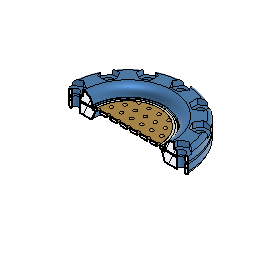
Microphone Capsule (Autodesk Fusion 360 design; units mm, degrees)
Autodesk Fusion 360 part; units mm, degrees
note: some values were not read from the file. Chosen so that the rebuilt part matches the saved one: which face or edge a step refers to. Set by a fixed rule: which sketch regions a step uses.
ref_plane "WorkPlane1" through (0, 0, -5) normal (0, 0, 1) x (1, 0, 0)
sketch "Top" plane through (0, 0, -5) normal (0, 0, 1) x (1, 0, 0)
  circle A0 centre (0, 0) radius 10.5
  circle A1 centre (0, 15.5) radius 1.175
  line L0 (0, 0) -> (0, 15.5) construction
  circle A2 centre (0, 0) radius 17.475
  circle A3 centre (0, 15.5) radius 1.975 construction
  circle A4 centre (-7.75, 13.4234) radius 1.175
  circle A5 centre (-13.4234, 7.75) radius 1.175
  circle A6 centre (-15.5, 0) radius 1.175
  circle A7 centre (-13.4234, -7.75) radius 1.175
  circle A8 centre (-7.75, -13.4234) radius 1.175
  circle A9 centre (0, -15.5) radius 1.175
  circle A10 centre (7.75, -13.4234) radius 1.175
  circle A11 centre (13.4234, -7.75) radius 1.175
  circle A12 centre (15.5, 0) radius 1.175
  circle A13 centre (13.4234, 7.75) radius 1.175
  circle A14 centre (7.75, 13.4234) radius 1.175
  circle A15 centre (0, 0) radius 11.4
  circle A16 centre (0, 0) radius 9.7
  line L1 (-1.1836, 13.45) -> (-2.3671, 15.5)
  line L2 (-2.3671, 15.5) -> (-1.1836, 17.55)
  line L3 (-1.1836, 17.55) -> (1.1836, 17.55)
  line L4 (1.1836, 17.55) -> (2.3671, 15.5)
  line L5 (2.3671, 15.5) -> (1.1836, 13.45)
  line L6 (-1.1836, 13.45) -> (1.1836, 13.45)
  circle A17 centre (0, 15.5) radius 2.05 construction
  line L7 (-7.75, 15.7905) -> (-5.7, 14.607)
  line L8 (-9.8, 14.607) -> (-7.75, 15.7905)
  line L9 (-9.8, 12.2398) -> (-9.8, 14.607)
  line L10 (-7.75, 11.0563) -> (-9.8, 12.2398)
  line L11 (-7.75, 11.0563) -> (-5.7, 12.2398)
  line L12 (-5.7, 14.607) -> (-5.7, 12.2398)
  line L13 (-14.607, 9.8) -> (-12.2398, 9.8)
  line L14 (-15.7905, 7.75) -> (-14.607, 9.8)
  line L15 (-14.607, 5.7) -> (-15.7905, 7.75)
  line L16 (-12.2398, 5.7) -> (-14.607, 5.7)
  line L17 (-12.2398, 5.7) -> (-11.0563, 7.75)
  line L18 (-12.2398, 9.8) -> (-11.0563, 7.75)
  line L19 (-17.55, 1.1836) -> (-15.5, 2.3671)
  line L20 (-17.55, -1.1836) -> (-17.55, 1.1836)
  line L21 (-15.5, -2.3671) -> (-17.55, -1.1836)
  line L22 (-13.45, -1.1836) -> (-15.5, -2.3671)
  line L23 (-13.45, -1.1836) -> (-13.45, 1.1836)
  line L24 (-15.5, 2.3671) -> (-13.45, 1.1836)
  line L25 (-15.7905, -7.75) -> (-14.607, -5.7)
  line L26 (-14.607, -9.8) -> (-15.7905, -7.75)
  line L27 (-12.2398, -9.8) -> (-14.607, -9.8)
  line L28 (-11.0563, -7.75) -> (-12.2398, -9.8)
  line L29 (-11.0563, -7.75) -> (-12.2398, -5.7)
  line L30 (-14.607, -5.7) -> (-12.2398, -5.7)
  line L31 (-9.8, -14.607) -> (-9.8, -12.2398)
  line L32 (-7.75, -15.7905) -> (-9.8, -14.607)
  line L33 (-5.7, -14.607) -> (-7.75, -15.7905)
  line L34 (-5.7, -12.2398) -> (-5.7, -14.607)
  line L35 (-5.7, -12.2398) -> (-7.75, -11.0563)
  line L36 (-9.8, -12.2398) -> (-7.75, -11.0563)
  line L37 (-1.1836, -17.55) -> (-2.3671, -15.5)
  line L38 (1.1836, -17.55) -> (-1.1836, -17.55)
  line L39 (2.3671, -15.5) -> (1.1836, -17.55)
  line L40 (1.1836, -13.45) -> (2.3671, -15.5)
  line L41 (1.1836, -13.45) -> (-1.1836, -13.45)
  line L42 (-2.3671, -15.5) -> (-1.1836, -13.45)
  line L43 (7.75, -15.7905) -> (5.7, -14.607)
  line L44 (9.8, -14.607) -> (7.75, -15.7905)
  line L45 (9.8, -12.2398) -> (9.8, -14.607)
  line L46 (7.75, -11.0563) -> (9.8, -12.2398)
  line L47 (7.75, -11.0563) -> (5.7, -12.2398)
  line L48 (5.7, -14.607) -> (5.7, -12.2398)
  line L49 (14.607, -9.8) -> (12.2398, -9.8)
  line L50 (15.7905, -7.75) -> (14.607, -9.8)
  line L51 (14.607, -5.7) -> (15.7905, -7.75)
  line L52 (12.2398, -5.7) -> (14.607, -5.7)
  line L53 (12.2398, -5.7) -> (11.0563, -7.75)
  line L54 (12.2398, -9.8) -> (11.0563, -7.75)
  line L55 (17.55, -1.1836) -> (15.5, -2.3671)
  line L56 (17.55, 1.1836) -> (17.55, -1.1836)
  line L57 (15.5, 2.3671) -> (17.55, 1.1836)
  line L58 (13.45, 1.1836) -> (15.5, 2.3671)
  line L59 (13.45, 1.1836) -> (13.45, -1.1836)
  line L60 (15.5, -2.3671) -> (13.45, -1.1836)
  line L61 (15.7905, 7.75) -> (14.607, 5.7)
  line L62 (14.607, 9.8) -> (15.7905, 7.75)
  line L63 (12.2398, 9.8) -> (14.607, 9.8)
  line L64 (11.0563, 7.75) -> (12.2398, 9.8)
  line L65 (11.0563, 7.75) -> (12.2398, 5.7)
  line L66 (14.607, 5.7) -> (12.2398, 5.7)
  line L67 (9.8, 14.607) -> (9.8, 12.2398)
  line L68 (7.75, 15.7905) -> (9.8, 14.607)
  line L69 (5.7, 14.607) -> (7.75, 15.7905)
  line L70 (5.7, 12.2398) -> (5.7, 14.607)
  line L71 (5.7, 12.2398) -> (7.75, 11.0563)
  line L72 (9.8, 12.2398) -> (7.75, 11.0563)
  circle A18 centre (0, 0) radius 10.6
  point P0 (0, 10.5)
  dimension "d2" = 21
  dimension "d3" = 2.35
  dimension "d7" = 0.8
  dimension "d9" = 360
  dimension "d35" = 4.1
  dimension "d62" = 0.8
  dimension "d63" = 0.1
  dimension "d82" = 5
  dimension "d83" = 0.8
  constraint coincident A0.centre L0.start
  constraint vertical L0
  constraint coincident A1.centre L0.end
  constraint concentric A0 A2
  constraint concentric A1 A3
  constraint tangent A2 A3
  constraint concentric A0 A15
  constraint perpendicular L0 L6
  constraint equal L5 L6
  constraint equal L4 L5
  constraint equal L3 L4
  constraint equal L2 L3
  constraint equal L1 L2
  constraint concentric A1 A17
  constraint tangent L5 A17
  constraint tangent L4 A17
  constraint tangent L3 A17
  constraint tangent L2 A17
  constraint tangent L1 A17
  constraint parallel L2 L5
  constraint concentric A16 A18
  constraint coincident A0 P0
  constraint coincident L0 P0
  measures "d2" diameter of A0
  measures "d3" diameter of A1
  measures "d7" distance of A1 A3
  measures "d35" distance of L2.end L6
  measures "d62" distance of A0 A16
  measures "d63" distance of A0 A18
  measures "d82" distance of A1.centre P0
  measures "d83" distance of A15 A18
ref_plane "WorkPlane2" through (0, -41, 0) normal (0, 1, 0) x (0, 0, 1)
sketch "Side" plane through (0, -41, 0) normal (0, 1, 0) x (1, 0, 0)
  line L0 (-17.475, 5) -> (17.475, 5)
  line L1 (-10.5, 5) -> (10.5, 5)
  line L2 (-11.4, 5) -> (11.4, 5)
  line L3 (17.475, -2.6) -> (17.475, -0.766)
  line L4 (17.475, -3.2) -> (10.75, -3.2)
  line L5 (12.95, -6.2) -> (16.475, -6.2)
  line L6 (17.475, -5.2) -> (17.475, -3.2)
  line L7 (17.475, 5) -> (17.475, 0) construction
  line L8 (10.5, 5) -> (10.5, -2.7) construction
  line L9 (17.1178, 0) -> (10.6827, 0)
  line L10 (10.6827, 0) -> (9.7, -2.7)
  line L11 (10.5, -3) -> (11.4, -3)
  line L12 (0, 0) -> (10.6827, 0) construction
  line L13 (0, 0) -> (0, 5) construction
  line L14 (-9.7, 5) -> (9.7, 5)
  line L15 (9.7, 5) -> (9.7, -2.7) construction
  line L16 (11.4, 5) -> (11.4, -3) construction
  line L17 (10.5, -3) -> (10.5, -2.7)
  line L18 (10.5, -2.7) -> (9.7, -2.7)
  line L19 (11.4, -3) -> (17.475, -3) construction
  line L20 (-10.6, 5) -> (10.6, 5)
  line L21 (10.6, 5) -> (10.6, -3.4598) construction
  line L22 (11.4, -3) -> (17.475, -2.6)
  arc A0 (16.475, -6.2) -> (17.475, -5.2) centre (16.475, -5.2) ccw
  arc A1 (17.475, -0.766) -> (17.1178, 0) centre (16.475, -0.766) ccw
  line L23 (17.1178, 0) -> (17.475, -0.2997) construction
  line L24 (17.475, -0.2997) -> (17.475, -0.766) construction
  line L25 (13.45, 5) -> (13.45, -6.2) construction
  arc A2 (10.75, -3.2) -> (10.6, -3.4598) centre (10.9, -3.4598) ccw
  arc A3 (10.6, -3.4598) -> (12.95, -6.2) centre (13.3726, -3.4598) ccw
  line L26 (10.75, -3.2) -> (10.6, -3.2866) construction
  point P0 (17.475, -6.2)
  point P1 (17.475, -2.6)
  point P2 (17.475, -4.6)
  point P3 (13.45, 5)
  point P4 (17.55, 5)
  dimension "d13" = 3
  dimension "d16" = 3
  dimension "d31" = 0.3
  dimension "d37" = 1.6
  dimension "d85" = 0.4
  dimension "d91" = 70
  dimension "d92" = 1
  dimension "d93" = 40
  dimension "d95" = 1
  dimension "d96" = 0.5
  dimension "d97" = 0.3
  dimension "d98" = 30
  dimension "d99" = 0.2
  constraint coincident L0.end L7.start
  constraint coincident L1.end L8.start
  constraint perpendicular L0 L8
  constraint perpendicular L0 L7
  constraint collinear L3 L6
  constraint collinear L3 L7
  constraint parallel L0 L9
  constraint parallel L9 L11
  constraint parallel L4 L11
  constraint coincident L12.start L13.start
  constraint collinear L9 L12
  constraint parallel L4 L5
  constraint midpoint L1 L13.end
  constraint coincident L14.end L15.start
  constraint perpendicular L0 L15
  constraint coincident L2.end L16.start
  constraint perpendicular L0 L16
  constraint perpendicular L11 L17
  constraint collinear L8 L17
  constraint coincident L6 P2
  constraint coincident L3 L19.end
  constraint perpendicular L3 L19
  constraint coincident L20.end L21.start
  constraint perpendicular L0 L21
  constraint coincident L8.end L17.end
  constraint coincident L7.end L9
  constraint coincident L7.end L3
  constraint coincident L3 P1
  constraint coincident P1 L22
  constraint coincident P0 L6
  constraint coincident P0 L5
  constraint tangent L6 A0
  constraint tangent L5 A0
  constraint coincident L9.end L10
  constraint coincident L10.start L9
  constraint coincident L10.end L15.end
  constraint parallel L9 L18
  constraint coincident L9.end L10.start
  constraint tangent L3 A1
  constraint coincident L9.start A1.end
  constraint tangent A1 L23
  constraint collinear L3 L24
  constraint coincident P3 L25.start
  constraint perpendicular L0 L25
  constraint coincident P1 L3.start
  constraint coincident L5 L25.end
  constraint tangent A2 A3
  constraint coincident L21.end A2.end
  constraint tangent L21 A3
  constraint coincident L4.end A2.start
  constraint tangent A2 L26
  constraint coincident L21 L26.end
  measures "d13" distance of L11.end L9
  measures "d16" distance of L4 P0
  measures "d31" distance of L11.start L8.end
  measures "d37" distance of L5 P2
  measures "d85" distance of L11 P1
  measures "d91" angle of L9 L10
  measures "d92" radius of A1
  measures "d93" angle of L9 L23
  measures "d95" radius of A0
  measures "d96" distance of L5.start L25
  measures "d97" radius of A2
  measures "d98" angle of L4 L26
  measures "d99" distance of L11 L4.end
ref_plane "WorkPlane3" through (0, 0, 0) normal (0, 1, 0) x (0, 0, 1)
sketch "Sketch3" plane through (0, 0, 0) normal (0, 1, 0) x (1, 0, 0)
  arc A0 (16.475, -6.2) -> (17.475, -5.2) centre (16.475, -5.2) ccw
  line L0 (12.95, -6.2) -> (16.475, -6.2)
  line L1 (17.475, -3.2) -> (10.75, -3.2)
  line L2 (17.475, -5.2) -> (17.475, -3.2)
  line L3 (17.475, -2.6) -> (17.475, -0.766)
  line L4 (11.4, -3) -> (17.475, -2.6)
  line L5 (10.5, -3) -> (11.4, -3)
  line L6 (10.5, -3) -> (10.5, -2.7)
  line L7 (10.5, -2.7) -> (9.7, -2.7)
  line L8 (10.6827, 0) -> (9.7, -2.7)
  line L9 (17.1178, 0) -> (10.6827, 0)
  arc A1 (17.475, -0.766) -> (17.1178, 0) centre (16.475, -0.766) ccw
  arc A2 (10.75, -3.2) -> (10.6, -3.4598) centre (10.9, -3.4598) ccw
  arc A3 (10.6, -3.4598) -> (12.95, -6.2) centre (13.3726, -3.4598) ccw
revolve "Revolve1" add sketch "Sketch3" angle 360 about axis through (0, 0, -4.7808) along (0, 0, 1) makes body 1 at (14.8693, -1.3812, 0) makes body 2 at (15.1283, -1.4022, 3.2)
extrude "Extrude3" cut sketch "Top" against normal up to surface (6.2 mm away) from surface at 11.2 contours A1 | A4 | A5 | A6 | A7 | A8 | A9 | A10 | A11 | A12 | A13 | A14 bodies 1 2
extrude "Extrude5" cut sketch "Top" against normal up to surface (1.6 mm away) from surface at 11.2 contours A2 L55 L57 L58 L59 L60 | A2 L55 L56 L57 | A2 L61 L63 L64 L65 L66 | A2 L61 L62 L63 | A2 L49 L50 L51 | A2 L49 L51 L52 L53 L54 | A2 L67 L69 L70 L71 L72 | A2 L67 L68 L69 | A2 L43 L44 L45 | A2 L43 L45 L46 L47 L48 | A2 L1 L2 L4 L5 L6 | A2 L2 L3 L4 | A2 L37 L38 L39 | A2 L37 L39 L40 L41 L42 | A2 L7 L9 L10 L11 L12 | A2 L7 L8 L9 | A2 L31 L32 L33 | A2 L31 L33 L34 L35 L36 | A2 L13 L15 L16 L17 L18 | A2 L13 L14 L15 | A2 L25 L26 L27 | A2 L25 L27 L28 L29 L30 | A2 L19 L21 L22 L23 L24 | A2 L19 L20 L21 bodies 2
ref_plane "WorkPlane1" through (0, 0, -10) normal (0, 0, 1) x (1, 0, 0) in component "Brass Base Plate"
sketch "Sketch1" plane through (0, 0, -10) normal (0, 0, 1) x (1, 0, 0) in component "Brass Base Plate"
  circle A0 centre (0, 0) radius 17.475 construction
  circle A1 centre (0, 0) radius 10.2
  line L0 (0, 10.2) -> (0, -10.2) construction
  arc A2 (-8.8335, 5.1) -> (8.8335, 5.1) centre (0, 10.2) ccw construction
  line L1 (8.8335, 5.1) -> (-8.8335, -5.1) construction
  line L2 (-8.8335, 5.1) -> (8.8335, -5.1) construction
  line L3 (0, 10.2) -> (8.8335, -5.1) construction
  line L4 (0, 10.2) -> (-8.8335, -5.1) construction
  line L5 (-9.8761, 2.55) -> (9.8761, 2.55) construction
  line L6 (8.8335, -5.1) -> (-8.8335, -5.1) construction
  line L7 (8.8335, 5.1) -> (0, -10.2) construction
  line L8 (9.9984, -2.0178) -> (3.2518, 9.6678) construction
  line L9 (-2.7297, 9.828) -> (7.1464, -7.278) construction
  circle A3 centre (4.4167, 2.55) radius 0.5
  circle A4 centre (5.889, 0) radius 0.5
  circle A5 centre (1.4722, 2.55) radius 0.5
  line L10 (9.9984, 2.0178) -> (3.2518, -9.6678) construction
  circle A6 centre (8.8335, 0) radius 0.5
  circle A7 centre (7.3612, 2.55) radius 0.5
  circle A8 centre (5.889, 5.1) radius 0.5
  circle A9 centre (4.4167, 7.65) radius 0.5
  circle A10 centre (2.9445, 5.1) radius 0.5
  circle A11 centre (-4.4167, 7.65) radius 0.5
  circle A12 centre (-1.4722, 7.65) radius 0.5
  circle A13 centre (-2.9445, 5.1) radius 0.5
  circle A14 centre (0, 5.1) radius 0.5
  circle A15 centre (1.4722, 7.65) radius 0.5
  circle A16 centre (4.4167, 7.65) radius 0.5
  circle A17 centre (2.9445, 5.1) radius 0.5
  circle A18 centre (-1.4722, 2.55) radius 0.5
  circle A19 centre (-8.8335, 0) radius 0.5
  circle A20 centre (-7.3612, 2.55) radius 0.5
  circle A21 centre (-5.889, 0) radius 0.5
  circle A22 centre (-4.4167, 2.55) radius 0.5
  circle A23 centre (-5.889, 5.1) radius 0.5
  circle A24 centre (-4.4167, 7.65) radius 0.5
  circle A25 centre (-2.9445, 5.1) radius 0.5
  circle A26 centre (-2.9445, 0) radius 0.5
  circle A27 centre (-4.4167, -7.65) radius 0.5
  circle A28 centre (-5.889, -5.1) radius 0.5
  circle A29 centre (-2.9445, -5.1) radius 0.5
  circle A30 centre (-4.4167, -2.55) radius 0.5
  circle A31 centre (-7.3612, -2.55) radius 0.5
  circle A32 centre (-8.8335, 0) radius 0.5
  circle A33 centre (-5.889, 0) radius 0.5
  circle A34 centre (-1.4722, -2.55) radius 0.5
  circle A35 centre (4.4167, -7.65) radius 0.5
  circle A36 centre (1.4722, -7.65) radius 0.5
  circle A37 centre (2.9445, -5.1) radius 0.5
  circle A38 centre (0, -5.1) radius 0.5
  circle A39 centre (-1.4722, -7.65) radius 0.5
  circle A40 centre (-4.4167, -7.65) radius 0.5
  circle A41 centre (-2.9445, -5.1) radius 0.5
  circle A42 centre (1.4722, -2.55) radius 0.5
  circle A43 centre (8.8335, 0) radius 0.5
  circle A44 centre (7.3612, -2.55) radius 0.5
  circle A45 centre (5.889, 0) radius 0.5
  circle A46 centre (4.4167, -2.55) radius 0.5
  circle A47 centre (5.889, -5.1) radius 0.5
  circle A48 centre (4.4167, -7.65) radius 0.5
  circle A49 centre (2.9445, -5.1) radius 0.5
  circle A50 centre (2.9445, 0) radius 0.5
  circle A51 centre (0, 0) radius 0.5
  point P0 (4.4167, 2.55)
  point P1 (-4.4167, 2.55)
  point P2 (7.3612, 2.55)
  point P3 (4.4167, -2.55)
  point P4 (5.889, -5.1)
  dimension "d45" = 20.4
  dimension "d64" = 1
  dimension "d66" = 360
  constraint concentric A0 A1
  constraint coincident A1 L0.start
  constraint coincident A1 L0.end
  constraint coincident A0.centre L0
  constraint vertical L0
  constraint coincident A0.centre A2
  constraint coincident A1 A2.start
  constraint coincident A1 A2.end
  constraint coincident L0.start A2.centre
  constraint coincident A1 L1.end
  constraint coincident A0.centre L1
  constraint coincident A1 L2.end
  constraint coincident A0.centre L2
  constraint coincident A1 L5.start
  constraint coincident A1 L5.end
  constraint coincident L1 P0
  constraint coincident L4 P1
  constraint coincident L2 P1
  constraint coincident L3 P0
  constraint coincident L5 P0
  constraint coincident L5 P1
  constraint coincident A1 L8.start
  constraint coincident A1 L8.end
  constraint perpendicular L1 L8
  constraint coincident L7 P2
  constraint coincident L5 P2
  constraint coincident L8 P2
  constraint coincident A1 L9.start
  constraint coincident A1 L9.end
  constraint coincident L7 P3
  constraint coincident L2 P3
  constraint coincident L9 P3
  constraint perpendicular L1 L9
  constraint coincident P0 A3.centre
  constraint coincident L3 A4.centre
  constraint coincident L7 A4.centre
  constraint coincident A1 L10.start
  constraint coincident A1 L10.end
  constraint coincident L6 P4
  constraint coincident L9 P4
  constraint coincident L10 P4
  constraint perpendicular L2 L10
  constraint coincident L10 A6.centre
  constraint coincident L8 A6.centre
  constraint coincident P2 A7.centre
  constraint equal A3 A7
  constraint equal A3 A4
  constraint equal A4 A6
  constraint equal A5 A6
  constraint symmetric L1 A4 A10
  constraint symmetric L1 A6 A9
  constraint symmetric L1 A7 A8
  constraint coincident A0.centre A1.centre
  constraint equal A5 A51
  constraint coincident L9 A5.centre
  constraint coincident L5 A5.centre
  measures "d45" diameter of A1
  measures "d64" diameter of A7
ref_plane "WorkPlane2" through (0, -46, 0) normal (0, 1, 0) x (0, 0, 1) in component "Brass Base Plate"
sketch "Sketch2" plane through (0, -46, 0) normal (0, 1, 0) x (1, 0, 0) in component "Brass Base Plate"
  line L0 (-10.2, 10) -> (10.2, 10)
  line L1 (10.2, -2.7) -> (-10.2, -2.7)
  line L2 (-10.2, -2.7) -> (-10.2, -3.1)
  arc A0 (-10.2, -3.1) -> (-9.8, -3.5) centre (-9.8, -3.1) ccw
  line L3 (-9.8, -3.5) -> (9.8, -3.5)
  arc A1 (9.8, -3.5) -> (10.2, -3.1) centre (9.8, -3.1) ccw
  line L4 (10.2, -3.1) -> (10.2, -2.7)
  arc A2 (10.2, -3.1) -> (9.8, -2.7) centre (9.8, -3.1) ccw construction
  line L5 (0, 10) -> (0, -2.7) construction
  arc A3 (9.8, -3.55) -> (10.2459, -3.0397) centre (9.8, -3.1) ccw
  line L6 (9.8, -3.55) -> (9.2, -3.55)
  line L7 (9.2, -3.55) -> (9.2, -3.5)
  line L8 (10.2459, -3.0397) -> (10.2, -2.7)
  point P0 (9.7, -2.7)
  dimension "d47" = 0.8
  dimension "d48" = 0.4
  dimension "d54" = 0.05
  dimension "d67" = 1
  constraint perpendicular L1 L2
  constraint tangent L2 A0
  constraint perpendicular L2 L3
  constraint perpendicular L1 L4
  constraint tangent A0 L3
  constraint tangent A1 L4
  constraint equal A0 A1
  constraint coincident L1 A2.end
  constraint coincident A1.end L4.start
  constraint tangent L1 A2
  constraint tangent L4 A2
  constraint equal A1 A2
  constraint parallel L0 L1
  constraint coincident P0 L1
  constraint midpoint L0 L5.start
  constraint midpoint L1 L5.end
  constraint perpendicular L0 L5
  constraint equal L0 L1
  constraint coincident L3 L7.end
  constraint perpendicular L3 L7
  constraint tangent A3 L6
  constraint tangent A3 L8
  constraint parallel L3 L6
  constraint tangent L3 A1
  constraint coincident A1.centre A2.centre
  measures "d47" distance of L1 L3.end
  measures "d48" radius of A1
  measures "d54" distance of L6.end L7.end
  measures "d67" distance of L4 L6.end
extrude "Extrude1" add sketch "Sketch1" along normal up to surface (0.8 mm away) from surface at 12.7 separate body makes body 3 in component "Brass Base Plate"
fillet "Fillet1" radius 0.4 1 edges at (-9.5097, 3.6885, 3.5) on bodies 3 in component "Brass Base Plate"
ref_plane "WorkPlane3" through (0, 0, 0) normal (0, 1, 0) x (0, 0, 1) in component "Brass Base Plate"
sketch "Sketch3 (2)" plane through (0, 0, 0) normal (0, 1, 0) x (1, 0, 0) in component "Brass Base Plate"
  line L0 (9.2, -3.55) -> (9.2, -3.5)
  line L1 (9.8, -3.55) -> (9.2, -3.55)
  arc A0 (9.8, -3.55) -> (10.2459, -3.0397) centre (9.8, -3.1) ccw
  line L2 (10.2459, -3.0397) -> (10.2, -2.7)
  arc A1 (9.8, -3.5) -> (10.2, -3.1) centre (9.8, -3.1) ccw
  line L3 (10.2, -3.1) -> (10.2, -2.7)
  line L4 (-9.8, -3.5) -> (9.8, -3.5)
  point P0 (9.2, -3.55)
revolve "Revolve1'" add sketch "Sketch3 (2)" angle 360 about axis through (0, 0, -10.7515) along (0, 0, 1) separate body makes body 4 in component "Brass Base Plate"
component "Brass Base Plate" placed x (1, 0, 0) y (0, 1, 0) z (0, 0, 1) at (0, 0, 0)
equation "d53 = d48"
named bodies: "MIC-CAP-P001D2", "MIC-CAP-P002D1"
